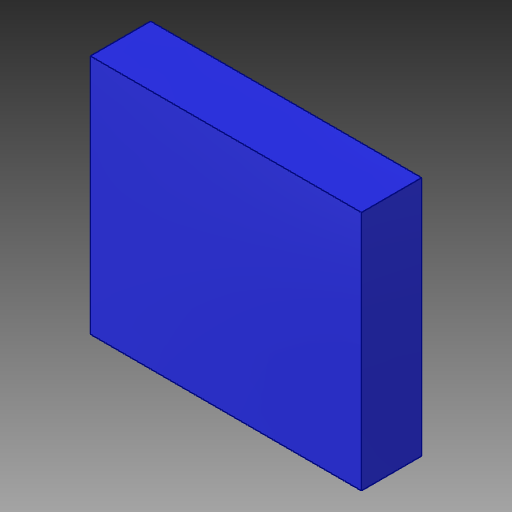
# Autodesk Inventor part: リング、スタート台2
Saved by Autodesk Inventor 2017 (Build 210142000, 142)
## iProperties
Part Number: リング、スタート台2
Material: 一般
Document SubType Name: Modeling
Designer: 雪村
Density: 1 g/cm^3
Appearance: 青 - 壁塗料 - 光沢
Mass: 18000 g
Surface Area: 5300 cm^2
Volume: 18000 cm^3
Author: 雪村
Autodesk Inventor part; units mm, degrees
ref_plane "YZ Plane" through (0, 0, 0) normal (1, 0, 0) x (0, 1, 0)
ref_plane "XZ Plane" through (0, 0, 0) normal (0, 1, 0) x (-1, 0, 0)
ref_plane "XY Plane" through (0, 0, 0) normal (0, 0, 1) x (1, 0, 0)
sketch "スケッチ1" plane through (0, 0, 0) normal (0, 0, 1) x (1, 0, 0)
  line L0 (0, 0) -> (450, 0)
  line L1 (450, 0) -> (450, 400)
  line L2 (450, 400) -> (0, 400)
  line L3 (0, 400) -> (0, 0)
  dimension "d0" = 450
  dimension "d1" = 400
  constraints: 8 end point, 2 horizontal, 2 vertical
  measures "d0" distance of L2.end L1.end
  measures "d1" distance of L1.end L0.end
extrude "押し出し1" add sketch "スケッチ1" along normal blind 100
